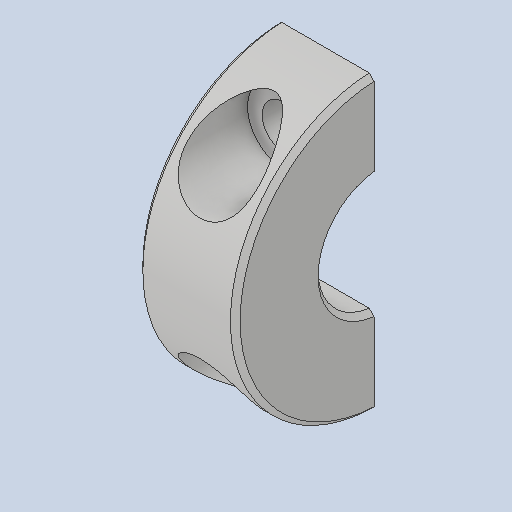
# Autodesk Inventor part: SSCSP12-10b
Saved by Autodesk Inventor 2025.2 (Build 292293000, 293)
## iProperties
Category: PARTsolutions
Company: MISUMI
Created: 2023-12-05
Part Number: SSCSP12-10b
Material: Generic
Catalog Web Link: www.cadenas.de
Description: SCSP,SCSPT,SCSPK,PSCSP,PSCSPT,PSCSPK,SSCSP,SCNPA,SCNPAW,SSCSPT,SSCSPK_b-Set Collars - Separate - Standard, 2 Taps (Coarse Thread), 2 Drill Hole Type
Vendor: MISUMI
Document SubType Name: Modeling
Designer: psAdmin
Manufacturer: MISUMI
Mass: 2.16407 g
Surface Area: 16.1745 cm^2
Volume: 2.16407 cm^3
Density: 1 g/cm^3
Appearance: PSOLRGB-191-191-191
PSOL_IDENT_0: {$CADENAS_DATA/23d-libs/misumi/metric/03_set_collars/scsp_b.prj},240 {VTYP=3D},{NB=SSCSP12-10b},{LIN
PSOL_IDENT_1: A=SSCSP12-10},{NN=SCSP,SCSPT,SCSPK,PSCSP,PSCSPT,PSCSPK,SSCSP,SCNPA,SCNPAW,SSCSPT,SSCSPK_b},{DATE=18.
PSOL_IDENT_2: 06.2021 05:38:29},{GEOMDATE=08.06.2021 04:15:22},{VERSION=},{LINEID=70},{WBVAR=TS,MAT,ST,BS},{WBNUME
PSOL_IDENT_3: RIC=BS}  {NB=SSCSP12-10b},{LINA=SSCSP12-10},{KT=DUMMY},{PN=SSCSP12-10},{TYPE=SSCSP},{TS=S},{MAT=304}
PSOL_IDENT_4: ,{ST=-},{AC=Hexagon Socket Head Cap Screws 2 Pcs. (SUS) },{D=12},{BS=10},{B1=8,10,12,15},{B2=8,10,12
PSOL_IDENT_5: },{BALG=8,10,12,15},{D1=30},{M=M4},{THMD=4},{ST0= '-','-' },{DD=4.5},{R=3.75},{W=1.5},{X=10.0},{Y=5.
PSOL_IDENT_6: 0},{M1=M4},{M1A=M4},{P1=22.0},{P11=22},{C=0.5},{L=12},{MATA=  '1045','S45C Equivalent','304','SUS304
PSOL_IDENT_7: Equivalent','2017','A2017(2017 Aluminum)(EN AW-2017_AlCu4MgSi)'   },{THMD1=4},{TS1= 'S', 'Standard'
PSOL_IDENT_8: ,'2H','2-Drill Hole','2T','2 Tapped' },{N=5.5},{N1=5.5},{P22=21.0},{P2=21.0},{COL=0.75,0.75,0.75,0.0
PSOL_IDENT_9: 0},{COLALG=1}
NB: SSCSP12-10b
NN: SCSP,SCSPT,SCSPK,PSCSP,PSCSPT,PSCSPK,SSCSP,SCNPA,SCNPAW,SSCSPT,SSCSPK_b
NT: Set Collars - Separate - Standard, 2 Taps (Coarse Thread), 2 Drill Hole Type
NBSYN: $PN.b
LINA: SSCSP12-10
CATALOG: Misumi
PN: SSCSP12-10
TS: Standard
MAT: SUS304 Equivalent
ST: -
AC: Hexagon Socket Head Cap Screws 2 Pcs. (SUS)
D: 12
BS: 10
DD: 4.5
W: 1.5
C: 0.5
SUPPLIER: MISUMI
ARTICLENO: SSCSP12-10b
BOMINFO: SSCSP12-10
CREATOR: CADENAS GmbH
d5: 0.000 mm
d6: 0.000 mm
Title: SSCSP12-10
Author: Cadenas PARTsolutions
Comments: Set Collars - Separate - Standard, 2 Taps (Coarse Thread), 2 Drill Hole Type
Autodesk Inventor part; units mm, degrees
sketch "Sketch_1" plane through (0, 0, 0) normal (0, 0, 1) x (1, 0, 0)
  line L0 (5, 0) -> (-5, 0)
  line L1 (-5, 14.5) -> (-5, 6.5)
  line L2 (-5, 6.5) -> (-4.5, 6)
  line L3 (-4.5, 6) -> (4.5, 6)
  line L4 (4.5, 6) -> (5, 6.5)
  line L5 (5, 6.5) -> (5, 14.5)
  line L6 (5, 14.5) -> (4.5, 15)
  line L7 (4.5, 15) -> (-4.5, 15)
  line L8 (-4.5, 15) -> (-5, 14.5)
  constraints: 18 end point
revolve "Revolution1" add sketch "Sketch_1" angle 180 about axis through (5, 0, 0) along (1, 0, 0)
sketch "Sketch_2" plane through (0, 0, 0) normal (1, 0, 0) x (0, 1, 0)
  line L0 (-15, 0.75) -> (-15, -0.75)
  line L1 (-15, -0.75) -> (15, -0.75)
  line L2 (15, -0.75) -> (15, 0.75)
  line L3 (15, 0.75) -> (-15, 0.75)
  constraints: 8 end point
extrude "Extrusion1" cut sketch "Sketch_2" along normal mid plane 10
sketch "Sketch_3" plane through (0, 0, 0) normal (1, 0, 0) x (0, 1, 0)
  line L0 (-10, 0) -> (-10, 15)
  line L1 (-10, 15) -> (-6.25, 15)
  line L2 (-6.25, 15) -> (-6.25, 5)
  line L3 (-6.25, 5) -> (-7.75, 5)
  line L4 (-7.75, 5) -> (-7.75, 0)
  line L5 (-7.75, 0) -> (-10, 0)
  line L6 (-10, 0) -> (-10, 15)
  constraints: 14 end point
revolve "Revolution2" cut sketch "Sketch_3" angle 360 about axis through (0, -10, 0) along (0, 0, -1)
sketch "Sketch_4" plane through (0, 0, 0) normal (1, 0, 0) x (0, 1, 0)
  line L0 (10, 0) -> (10, 15)
  line L1 (10, 15) -> (13.75, 15)
  line L2 (13.75, 15) -> (13.75, 5)
  line L3 (13.75, 5) -> (12.25, 5)
  line L4 (12.25, 5) -> (12.25, 0)
  line L5 (12.25, 0) -> (10, 0)
  line L6 (10, 0) -> (10, 15)
  constraints: 14 end point
revolve "Revolution3" cut sketch "Sketch_4" angle 360 about axis through (0, 10, 0) along (0, 0, -1)
ref_plane "1_2_XY" through (0, 0, 0) normal (0, 0, 1) x (1, 0, 0)
ref_plane "1_2_YZ" through (0, 0, 0) normal (1, 0, 0) x (0, 1, 0)
ref_plane "1_2_ZX" through (0, 0, 0) normal (0, 1, 0) x (0, 0, 1)
ref_plane "body_screw_XY" through (0, -10, 5) normal (0, 0, 1) x (1, 0, 0)
ref_plane "body_screw_YZ" through (0, -10, 5) normal (1, 0, 0) x (0, 1, 0)
ref_plane "body_screw_ZX" through (0, -10, 5) normal (0, 1, 0) x (0, 0, 1)
ref_plane "body_screw2_XY" through (0, 10, 5) normal (0, 0, 1) x (1, 0, 0)
ref_plane "body_screw2_YZ" through (0, 10, 5) normal (1, 0, 0) x (0, 1, 0)
ref_plane "body_screw2_ZX" through (0, 10, 5) normal (0, 1, 0) x (0, 0, 1)
body "Solid1"
